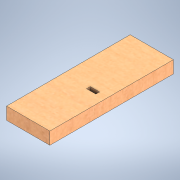
# Autodesk Inventor part: floor_side
Saved by Autodesk Inventor 2021 (Build 250183000, 183)
## iProperties
Created: 2020-06-13
Part Number: floor_side
Material: Generic
Document SubType Name: Modeling
Designer: Yatekii
Density: 1 g/cm^3
Appearance: Default
Author: Yatekii
Autodesk Inventor part; units mm, degrees
ref_plane "YZ Plane" through (0, 0, 0) normal (1, 0, 0) x (0, 1, 0)
ref_plane "XZ Plane" through (0, 0, 0) normal (0, 1, 0) x (-1, 0, 0)
ref_plane "XY Plane" through (0, 0, 0) normal (0, 0, 1) x (1, 0, 0)
sketch "Sketch1" plane through (0, 0, 0) normal (0, 1, 0) x (-1, 0, 0)
  line L0 (-17.5, -50) -> (17.5, -50)
  line L1 (17.5, -50) -> (17.5, 50)
  line L2 (17.5, 50) -> (-17.5, 50)
  line L3 (-17.5, 50) -> (-17.5, -50)
  line L4 (-17.5, -50) -> (17.5, 50) construction
  line L5 (17.5, -50) -> (-17.5, 50) construction
  point P0 (0, 0)
  dimension "d0" = 35
  dimension "d1" = 100
  constraints: 12 end point, 2 midpoint, 2 parallel, 1 horizontal, 1 perpendicular
  measures "d0" distance of L2.end L1.end
  measures "d1" distance of L1.end L0.end
extrude "Extrusion1" add sketch "Sketch1" along normal blind 10
sketch "Sketch3" plane through (0, 10, 0) normal (0, 1, 0) x (1, 0, 0)
  line L0 (2.75, -5.5) -> (10.25, -5.5)
  line L1 (10.25, -5.5) -> (10.25, -2.5)
  line L2 (10.25, -2.5) -> (2.75, -2.5)
  line L3 (2.75, -2.5) -> (2.75, -5.5)
  line L4 (2.75, -5.5) -> (10.25, -2.5) construction
  line L5 (10.25, -5.5) -> (2.75, -2.5) construction
  line L6 (-17.5, 50) -> (-17.5, -50) projected
  line L7 (-24.5, 0) -> (24.5, 0) projected
  line L8 (17.5, -50) -> (17.5, 50) projected
  point P0 (0, 0)
  point P1 (6.5, 0)
  point P2 (6.5, 0)
  point P3 (6.5, -4)
  dimension "d11" = 7.5
  dimension "d14" = 7.25
  dimension "d15" = 3
  dimension "d17" = 2.5
  constraints: 12 end point, 2 parallel, 1 horizontal, 1 midpoint, 1 perpendicular, 1 point on line
  measures "d11" distance of L0.start L0.end
  measures "d14" distance between parallel lines of L8 L1
  measures "d15" distance of L0.end L1.end
  measures "d17" distance between parallel lines of L7 L2
extrude "Extrusion3" cut sketch "Sketch3" against normal blind 10
body "Solid1"
